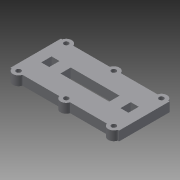
# Autodesk Inventor part: Top Clamp 6_6
Saved by Autodesk Inventor 2016 (Build 200138000, 138)
## iProperties
Created: 2015-05-18
Part Number: Top Clamp 6_6
Material: Generic
Document SubType Name: Modeling
Designer: Jonathan
Density: 1 g/cm^3
Appearance: Default
Mass: 56.079 g
Surface Area: 178.598 cm^2
Volume: 56.079 cm^3
Author: Jonathan
Autodesk Inventor part; units mm, degrees
ref_plane "YZ Plane" through (0, 0, 0) normal (1, 0, 0) x (0, 1, 0)
ref_plane "XZ Plane" through (0, 0, 0) normal (0, 1, 0) x (-1, 0, 0)
ref_plane "XY Plane" through (0, 0, 0) normal (0, 0, 1) x (1, 0, 0)
sketch "Sketch1" plane through (0, 0, 0) normal (0, 1, 0) x (-1, 0, 0)
  line L0 (58, 27) -> (-58, 27)
  line L1 (-58, 27) -> (-58, -27)
  line L2 (-58, -27) -> (58, -27)
  line L3 (58, -27) -> (58, 27)
  line L4 (58, 27) -> (-58, -27) construction
  line L5 (-58, 27) -> (58, -27) construction
  point P0 (0, 0)
  dimension "d0" = 116
  dimension "d1" = 54
  constraints: 12 end point, 2 midpoint, 2 parallel, 1 horizontal, 1 perpendicular
  measures "d0" distance of L2.end L1.end
  measures "d1" distance of L2.end L0.start
extrude "Body" add sketch "Sketch1" along normal mid plane 10
sketch "Sketch12" plane through (0, 5, 0) normal (0, 1, 0) x (1, 0, 0)
  line L0 (58, 27) -> (-58, 27) projected
  circle A0 centre (-50.8, 25.4) radius 6
  line L1 (-58, -27) -> (-58, 27) projected
  line L2 (-58, 0) -> (58, 0)
  line L3 (58, 27) -> (58, -27) projected
  line L4 (-58, -27) -> (58, -27) projected
  line L5 (0, -27) -> (0, 27)
  circle A1 centre (50.8, 25.4) radius 6
  circle A2 centre (-50.8, -25.4) radius 6
  circle A3 centre (50.8, -25.4) radius 6
  line L6 (-50.8, 25.4) -> (50.8, 25.4)
  line L7 (-50.8, -25.4) -> (50.8, -25.4)
  circle A4 centre (0, 25.4) radius 6
  circle A5 centre (0, -25.4) radius 6
  point P0 (0, 0)
  dimension "d40" = 25.4
  dimension "d49" = 50.8
  dimension "d57" = 12
  constraints: 8 end point, 6 centre point, 5 midpoint, 4 symmetric about line, 1 equal radius, 1 horizontal, 1 parallel, 4 other
  measures "d40" distance from line of L6.start L2
  measures "d49" horizontal distance of L5.end L6.start
  measures "d57" diameter of A4
extrude "Screw clamp boss" add sketch "Sketch12" against normal up to surface (10 mm away) contours A1 L0 | L0 A1 | A4 L6 L5 L0 | L0 A4 | A5 L7 L5 | L5 L7 A5 | A4 L6 L5 | L5 L6 A4 | A3 L4 | L4 A3 | L5 L6 A4 L0 | L7 A5 L4 L5 | L5 L4 A5 L7 | A0 L0 | L0 A0 | A2 L4 | L4 A2 | L4 A5
sketch "Sketch15" plane through (0, 5, 0) normal (0, 1, 0) x (1, 0, 0)
  circle A0 centre (0, 25.4) radius 2.55
  arc A1 (5.7827, 27) -> (-5.7827, 27) centre (0, 25.4) ccw projected
  circle A2 centre (-50.8, 25.4) radius 2.55
  arc A3 (-45.0173, 27) -> (-56.5827, 27) centre (-50.8, 25.4) ccw projected
  line L0 (55.75, -18.75) -> (-55.75, -18.75) projected
  line L1 (0, -18.75) -> (0, 18.75)
  line L2 (-55.75, 18.75) -> (55.75, 18.75) projected
  line L3 (-58, 27) -> (-58, -27) projected
  line L4 (-58, 0) -> (58, 0)
  line L5 (58, -27) -> (58, 27) projected
  circle A4 centre (50.8, 25.4) radius 2.55
  circle A5 centre (0, -25.4) radius 2.55
  circle A6 centre (-50.8, -25.4) radius 2.55
  circle A7 centre (50.8, -25.4) radius 2.55
  point P0 (0, 0)
  dimension "d60" = 5.1
  constraints: 6 centre point, 4 end point, 4 midpoint, 4 symmetric about line, 2 concentric, 1 equal radius, 4 other
  measures "d60" diameter of A0
extrude "Screw Clamp Hole" cut sketch "Sketch15" against normal through all
sketch "Sketch17" plane through (0, 5, 0) normal (0, 1, 0) x (1, 0, 0)
  line L0 (-46.5, -5.5) -> (46.5, -5.5)
  line L1 (46.5, -5.5) -> (46.5, 5.5)
  line L2 (46.5, 5.5) -> (-46.5, 5.5)
  line L3 (-46.5, 5.5) -> (-46.5, -5.5)
  line L4 (-46.5, -5.5) -> (46.5, 5.5) construction
  line L5 (46.5, -5.5) -> (-46.5, 5.5) construction
  line L6 (-38, -5.5) -> (-26, -5.5)
  line L7 (-26, -5.5) -> (-26, 5.5)
  line L8 (-26, 5.5) -> (-38, 5.5)
  line L9 (-38, 5.5) -> (-38, -5.5)
  arc A0 (-5.7827, -27) -> (5.7827, -27) centre (0, -25.4) ccw projected
  circle A1 centre (0, 25.4) radius 2.55 projected
  line L10 (0, -25.4) -> (0, 25.4)
  line L11 (26, -5.5) -> (38, -5.5)
  line L12 (38, -5.5) -> (38, 5.5)
  line L13 (38, 5.5) -> (26, 5.5)
  line L14 (26, 5.5) -> (26, -5.5)
  point P0 (0, 0)
  dimension "d70" = 93
  dimension "d71" = 11
  dimension "d72" = 38
  dimension "d73" = 12
  constraints: 30 end point, 6 parallel, 4 point on line, 3 horizontal, 3 perpendicular, 2 midpoint, 1 vertical, 2 other
  measures "d70" distance of L2.end L1.end
  measures "d71" distance of L1.end L0.end
  measures "d72" distance from line of point (0, 0) L9
  measures "d73" distance between parallel lines of L7 L9
extrude "Main Window" cut sketch "Sketch17" against normal through all contours L7 L2 L10 L0 | L10 L2 L14 L0
sketch "Sketch18" plane through (0, 5, 0) normal (0, 1, 0) x (1, 0, 0)
  line L0 (-46.5, -5.5) -> (46.5, -5.5)
  line L1 (46.5, -5.5) -> (46.5, 5.5)
  line L2 (46.5, 5.5) -> (-46.5, 5.5)
  line L3 (-46.5, 5.5) -> (-46.5, -5.5)
  line L4 (-46.5, -5.5) -> (46.5, 5.5) construction
  line L5 (46.5, -5.5) -> (-46.5, 5.5) construction
  line L6 (-38, -5.5) -> (-26, -5.5)
  line L7 (-26, -5.5) -> (-26, 5.5)
  line L8 (-26, 5.5) -> (-38, 5.5)
  line L9 (-38, 5.5) -> (-38, -5.5)
  arc A0 (-5.7827, -27) -> (5.7827, -27) centre (0, -25.4) ccw
  circle A1 centre (0, 25.4) radius 2.55
  line L10 (0, -25.4) -> (0, 25.4)
  line L11 (26, -5.5) -> (38, -5.5)
  line L12 (38, -5.5) -> (38, 5.5)
  line L13 (38, 5.5) -> (26, 5.5)
  line L14 (26, 5.5) -> (26, -5.5)
  point P0 (0, 0)
  point P1 (0, 0)
  dimension "d76" = 93
  dimension "d77" = 11
  dimension "d78" = 38
  dimension "d79" = 12
  constraints: 30 end point, 6 parallel, 4 point on line, 3 horizontal, 3 perpendicular, 2 centre point, 2 midpoint, 2 point on circle, 1 vertical, 2 other
  measures "d76" distance of L2.end L1.end
  measures "d77" distance of L1.end L0.end
  measures "d78" distance from line of point (0, 0) L9
  measures "d79" distance between parallel lines of L7 L9
extrude "Inelt Outlet Access" cut sketch "Sketch18" against normal through all contours L3 L2 L9 L0 | L12 L2 L1 L0
body "Solid1"
